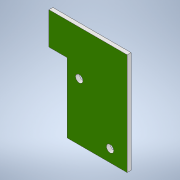
# Autodesk Inventor part: PCB_2_Miras
Saved by Autodesk Inventor 2022 (Build 260153000, 153)
## iProperties
Created: 2023-01-03
Part Number: PCB_2_Miras
Material: Generic
Document SubType Name: Modeling
Designer: Kamil
Density: 1 g/cm^3
Appearance: Default
Author: Kamil
Autodesk Inventor part; units mm, degrees
ref_plane "YZ Plane" through (0, 0, 0) normal (1, 0, 0) x (0, 1, 0)
ref_plane "XZ Plane" through (0, 0, 0) normal (0, 1, 0) x (-1, 0, 0)
ref_plane "XY Plane" through (0, 0, 0) normal (0, 0, 1) x (1, 0, 0)
sketch "Sketch1" plane through (0, 0, 0) normal (0, 0, 1) x (1, 0, 0)
  line L0 (12.5, -5.24) -> (15, -5.24) projected
  line L1 (15, -5.24) -> (15, -10.24) projected
  line L2 (15, -10.24) -> (12.5, -10.24) projected
  arc A0 (12.5, -5.24) -> (12.5, -10.24) centre (12.5, -7.74) ccw projected
  line L3 (-15, -5.24) -> (-12.5, -5.24) projected
  arc A1 (-12.5, -10.24) -> (-12.5, -5.24) centre (-12.5, -7.74) ccw projected
  line L4 (-12.5, -10.24) -> (-15, -10.24) projected
  line L5 (-15, -10.24) -> (-15, -5.24) projected
  circle A2 centre (-7.5, -12.2) radius 1.75 projected
  circle A3 centre (7.5, -12.2) radius 1.75 projected
  line L6 (-37.5, 12.4539) -> (-37.5, -12.4) projected
  line L7 (-34.5, -15.4) -> (34.5, -15.4) projected
  line L8 (37.5, -12.4) -> (37.5, 15.1772) projected
  line L9 (17.8602, 10.1005) -> (17.8602, -0.2) projected
  line L10 (14.8602, -3.2) -> (12.1354, -3.2) projected
  line L11 (10.655, -3.5907) -> (7.417, -5.4279) projected
  line L12 (5.9366, -5.8186) -> (-5.9366, -5.8186) projected
  line L13 (-7.417, -5.4279) -> (-10.655, -3.5907) projected
  line L14 (-12.1354, -3.2) -> (-14.8602, -3.2) projected
  line L15 (-17.8602, -0.2) -> (-17.8602, 10.3433) projected
  line L16 (-13.55, 20.254) -> (-13.55, 16.1005) projected
  line L17 (2.4, 23.254) -> (-10.55, 23.254) projected
  line L18 (2.4, 25.954) -> (2.4, 23.254) projected
  line L19 (4, 25.954) -> (2.4, 25.954) projected
  line L20 (4, 23.254) -> (4, 25.954) projected
  line L21 (5.95, 23.254) -> (4, 23.254) projected
  line L22 (8.95, 16.1005) -> (8.95, 20.254) projected
  line L23 (14.8602, 13.1005) -> (11.95, 13.1005) projected
  line L24 (50, 22.6643) -> (44, 22.6643) projected
  line L25 (44, 22.6643) -> (44, -4.7413) projected
  arc A4 (44, -9.7413) -> (44, -4.7413) centre (44, -7.2413) ccw projected
  line L26 (44, -9.7413) -> (44, -18.8012) projected
  line L27 (44, -18.8012) -> (50, -18.8012) projected
  line L28 (50, -18.8012) -> (50, 22.6643) projected
  line L29 (40.2471, -8.6254) -> (44, -18.8012) projected
  line L30 (44, -9.7413) -> (44, -18.8012) projected
  arc A5 (44, -4.7413) -> (44, -9.7413) centre (44, -7.2413) ccw projected
  line L31 (44, 4.3187) -> (44, -4.7413) projected
  line L32 (44, 4.3187) -> (40.2471, -5.8572) projected
  arc A6 (40.2471, -5.8572) -> (40.2471, -8.6254) centre (44, -7.2413) ccw projected
  line L33 (8.95, 13.1005) -> (37.5, 13.1005)
  line L34 (37.5, 13.1005) -> (37.5, 31.0066)
  line L35 (37.5, 31.0066) -> (8.95, 31.0066)
  line L36 (8.95, 31.0066) -> (8.95, 13.1005)
  line L37 (44, 18.1772) -> (41, 18.1772)
  line L38 (41, 18.1772) -> (41, 7.8033)
  line L39 (41, 7.8033) -> (44, 7.8033)
  line L40 (44, 7.8033) -> (44, 18.1772)
  line L41 (37.5, 31.0066) -> (41, 31.0066)
  line L42 (41, 31.0066) -> (41, 1.9316)
  line L43 (41, 1.9316) -> (37.5, 1.9316)
  line L44 (37.5, 1.9316) -> (37.5, 31.0066)
  line L45 (8.95, 31.0066) -> (41, 31.0066)
  line L46 (41, 31.0066) -> (41, 23.254)
  line L47 (41, 23.254) -> (8.95, 23.254)
  line L48 (8.95, 23.254) -> (8.95, 31.0066)
  line L49 (17.8602, 13.1005) -> (37.5, 13.1005)
  line L50 (37.5, 13.1005) -> (37.5, -15.4)
  line L51 (37.5, -15.4) -> (17.8602, -15.4)
  line L52 (17.8602, -15.4) -> (17.8602, 13.1005)
  line L53 (37.5, -15.4) -> (41, -15.4)
  line L54 (41, -15.4) -> (41, 1.9316)
  line L55 (41, 1.9316) -> (37.5, 1.9316)
  line L56 (37.5, 1.9316) -> (37.5, -15.4)
  arc A7 (-17.7252, -6.9095) -> (-17.704, -4.5096) centre (-17.7146, -5.7096) ccw projected
  line L57 (-17.7252, -6.9095) -> (-18.8252, -6.8998) projected
  arc A8 (-18.8039, -4.4999) -> (-18.8252, -6.8998) centre (-18.8145, -5.6998) ccw projected
  line L58 (-18.8039, -4.4999) -> (-17.704, -4.5096) projected
  circle A9 centre (21.3634, 8.1005) radius 1.5 projected
  arc A10 (-17.5172, 16.5895) -> (-17.496, 18.9894) centre (-17.5066, 17.7895) ccw projected
  line L59 (-17.5172, 16.5895) -> (-18.6172, 16.5993) projected
  arc A11 (-18.5959, 18.9992) -> (-18.6172, 16.5993) centre (-18.6065, 17.7992) ccw projected
  line L60 (-18.5959, 18.9992) -> (-17.496, 18.9894) projected
  circle A12 centre (34, -10.4) radius 1.5 projected
  arc A13 (34.5, -15.4) -> (37.5, -12.4) centre (34.5, -12.4) ccw projected
  arc A14 (37.5, 15.1772) -> (34.5, 18.1772) centre (34.5, 15.1772) ccw projected
  line L61 (34.5, 18.1772) -> (16.4051, 18.1772) projected
  arc A15 (13.4051, 21.1772) -> (16.4051, 18.1772) centre (16.4051, 21.1772) ccw projected
  line L62 (13.4051, 21.1772) -> (13.4051, 28.0066) projected
  arc A16 (13.4051, 28.0066) -> (10.4051, 31.0066) centre (10.4051, 28.0066) ccw projected
  line L63 (10.4051, 31.0066) -> (-18.5665, 31.0066) projected
  arc A17 (-18.5665, 31.0066) -> (-21.5665, 28.0066) centre (-18.5665, 28.0066) ccw projected
  line L64 (-21.5665, 28.0066) -> (-21.5665, 18.4539) projected
  arc A18 (-24.5665, 15.4539) -> (-21.5665, 18.4539) centre (-24.5665, 18.4539) ccw projected
  line L65 (-24.5665, 15.4539) -> (-34.5, 15.4539) projected
  arc A19 (-34.5, 15.4539) -> (-37.5, 12.4539) centre (-34.5, 12.4539) ccw projected
  arc A20 (-37.5, -12.4) -> (-34.5, -15.4) centre (-34.5, -12.4) ccw projected
  arc A21 (-10.655, -3.5907) -> (-12.1354, -3.2) centre (-12.1354, -6.2) ccw projected
  arc A22 (-17.8602, -0.2) -> (-14.8602, -3.2) centre (-14.8602, -0.2) ccw projected
  arc A23 (-15.7051, 13.2219) -> (-17.8602, 10.3433) centre (-14.8602, 10.3433) ccw projected
  arc A24 (-15.7051, 13.2219) -> (-13.55, 16.1005) centre (-16.55, 16.1005) ccw projected
  arc A25 (-10.55, 23.254) -> (-13.55, 20.254) centre (-10.55, 20.254) ccw projected
  arc A26 (8.95, 20.254) -> (5.95, 23.254) centre (5.95, 20.254) ccw projected
  arc A27 (8.95, 16.1005) -> (11.95, 13.1005) centre (11.95, 16.1005) ccw projected
  arc A28 (17.8602, 10.1005) -> (14.8602, 13.1005) centre (14.8602, 10.1005) ccw projected
  arc A29 (14.8602, -3.2) -> (17.8602, -0.2) centre (14.8602, -0.2) ccw projected
  arc A30 (12.1354, -3.2) -> (10.655, -3.5907) centre (12.1354, -6.2) ccw projected
  arc A31 (5.9366, -5.8186) -> (7.417, -5.4279) centre (5.9366, -2.8186) ccw projected
  arc A32 (-7.417, -5.4279) -> (-5.9366, -5.8186) centre (-5.9366, -2.8186) ccw projected
  point P0 (0, 0)
  point P1 (41, -3.8157)
  point P2 (41, -10.6668)
  point P3 (10.4051, 31.0066)
  dimension "d0" = 3
  constraints: 48 end point, 12 parallel, 6 horizontal, 6 perpendicular, 2 point on line
  measures "d0" distance of L39.end L38.end
extrude "Extrusion1" add sketch "Sketch1" along normal blind 3.1 contours L52 L9 L33 L8 A13 L7 | A28 L33 L52 | L8 L34 L47 L42 L38 L43 | L33 L23 A27 L22 L36 L47 L62 A15 L61 A14 L8 | L35 A16 L62 L47 L36 | L33 L36 A27 | L41 L42 L47 L34 | A9 | A12
sketch "Sketch2" plane through (0, 0, 0) normal (0, 0, -1) x (-1, 0, 0)
  line L0 (-17.8602, -15.4) -> (-34.5, -15.4) projected
  line L1 (-17.8602, 10.1005) -> (-17.8602, -15.4) projected
  line L2 (-8.95, 13.1005) -> (-14.8602, 13.1005) projected
  line L3 (-8.95, 31.0066) -> (-8.95, 13.1005) projected
  line L4 (-41, 1.9316) -> (-41, 31.0066) projected
  arc A0 (-16.4051, 18.1772) -> (-13.4051, 21.1772) centre (-16.4051, 21.1772) ccw projected
  line L5 (-34.5, 18.1772) -> (-16.4051, 18.1772) projected
  arc A1 (-34.5, 18.1772) -> (-37.5, 15.1772) centre (-34.5, 15.1772) ccw projected
  line L6 (-37.5, 31.0066) -> (-37.5, 15.1772) projected
  line L7 (-41, 31.0066) -> (-37.5, 31.0066) projected
  line L8 (-37.5, 1.9316) -> (-41, 1.9316) projected
  line L9 (-37.5, -12.4) -> (-37.5, 1.9316) projected
  arc A2 (-37.5, -12.4) -> (-34.5, -15.4) centre (-34.5, -12.4) ccw projected
  arc A3 (-14.8602, 13.1005) -> (-17.8602, 10.1005) centre (-14.8602, 10.1005) ccw projected
  line L10 (-10.4051, 31.0066) -> (-8.95, 31.0066) projected
  arc A4 (-10.4051, 31.0066) -> (-13.4051, 28.0066) centre (-10.4051, 28.0066) ccw projected
  line L11 (-13.4051, 21.1772) -> (-13.4051, 28.0066) projected
  point P0 (0, 0)
extrude "Extrusion2" cut sketch "Sketch2" against normal blind 1.5
sketch "Sketch3" plane through (41, -3.8157, 3.1) normal (1, 0, 0) x (0, 0, -1)
  line L0 (38.317, 76.7923) -> (28.0867, 64.6003) projected
  line L1 (-3.9, -14.9855) -> (-3.9, 26.48) projected
  line L2 (-3.9, -14.9855) -> (7.1, -14.9855) projected
  line L3 (7.1, -14.9855) -> (7.1, 1.1145) projected
  arc A0 (25.2, 19.2145) -> (7.1, 1.1145) centre (25.2, 1.1145) ccw projected
  line L4 (25.2, 19.2145) -> (36.2, 19.2145) projected
  line L5 (1.6, 5.7473) -> (1.6, 34.8223) projected
  line L6 (1.6, 34.8223) -> (0, 34.8223) projected
  line L7 (0, 5.7473) -> (0, 34.8223) projected
  line L8 (0, 0) -> (0, 34.8223) projected
  line L9 (0, 30.197) -> (1.6, 30.197)
  line L10 (28.0867, 30.906) -> (23.6867, 30.906) projected
  line L11 (23.6867, 30.906) -> (23.6867, 44.6714) projected
  line L12 (23.6867, 44.6714) -> (28.0867, 44.6714) projected
  line L13 (28.0867, 44.6714) -> (28.0867, 30.906) projected
  line L14 (28.0867, 64.6003) -> (28.0867, 59.2448) projected
  line L15 (36.2, 19.2145) -> (36.2, 63.075) projected
  line L16 (36.2, 63.075) -> (39.2, 63.075) projected
  line L17 (39.2, 63.075) -> (39.2, 76.4709) projected
  line L18 (23.5929, 59.2448) -> (-3.9, 26.48) projected
  arc A1 (39.2, 76.4709) -> (38.317, 76.7923) centre (38.7, 76.4709) ccw projected
  line L19 (23.5929, 59.2448) -> (28.0867, 59.2448) projected
  line L20 (11.8485, 39.6478) -> (14.4531, 37.4623) projected
  line L21 (14.4531, 37.4623) -> (10.9819, 33.3255) projected
  line L22 (10.9819, 33.3255) -> (8.3773, 35.511) projected
  line L23 (11.8485, 39.6478) -> (8.3773, 35.511) projected
  line L24 (1.6, 5.7473) -> (0, 5.7473) projected
  point P0 (3.1, 3.8157)
  point P1 (36.2, 74.2694)
  constraints: 2 end point, 2 point on line, 1 perpendicular
extrude "Extrusion3" cut sketch "Sketch3" against normal through all contours L18 L7 L6 L5 | L5 L9 L7 L18
sketch "Sketch4" plane through (0, 0, 3.1) normal (0, 0, 1) x (1, 0, 0)
  line L0 (31.7, -15.7) -> (31.7, 9.3) projected
  line L1 (13.4051, 26.3813) -> (8.95, 26.3813) projected
  line L2 (8.95, 26.3813) -> (8.95, 13.1005) projected
  line L3 (8.95, 13.1005) -> (14.8602, 13.1005) projected
  line L4 (17.8602, 10.1005) -> (17.8602, -15.4) projected
  line L5 (17.8602, -15.4) -> (34.5, -15.4) projected
  line L6 (41, 1.9316) -> (41, 26.3813) projected
  line L7 (41, -15.4) -> (41, -10.6668) projected
  line L8 (41, -3.8157) -> (41, -10.6668)
  arc A0 (17.8602, 10.1005) -> (14.8602, 13.1005) centre (14.8602, 10.1005) ccw projected
  arc A1 (34.5, -15.4) -> (37.5, -12.4) centre (34.5, -12.4) ccw projected
  line L9 (37.5, -12.4) -> (37.5, 1.9316) projected
  line L10 (37.5, 1.9316) -> (41, 1.9316) projected
  line L11 (41, 26.3813) -> (37.5, 26.3813) projected
  line L12 (37.5, 26.3813) -> (37.5, 15.1772) projected
  arc A2 (37.5, 15.1772) -> (34.5, 18.1772) centre (34.5, 15.1772) ccw projected
  line L13 (34.5, 18.1772) -> (16.4051, 18.1772) projected
  arc A3 (13.4051, 21.1772) -> (16.4051, 18.1772) centre (16.4051, 21.1772) ccw projected
  line L14 (13.4051, 21.1772) -> (13.4051, 26.3813) projected
  point P0 (0, 0)
  constraints: 2 end point
extrude "Extrusion4" [suppressed]
sketch "Sketch5" plane through (0, 0, 3.1) normal (0, 0, 1) x (1, 0, 0)
  line L0 (13.4051, 26.3813) -> (8.95, 26.3813) projected
  line L1 (8.95, 26.3813) -> (8.95, 13.1005) projected
  line L2 (8.95, 13.1005) -> (14.8602, 13.1005) projected
  line L3 (17.8602, 10.1005) -> (17.8602, -15.4) projected
  line L4 (17.8602, -15.4) -> (34.5, -15.4) projected
  line L5 (15, 8.3373) -> (15, -1.2152) projected
  line L6 (8.95, 13.1005) -> (17.8602, 13.1005) projected
  line L7 (17.8602, 13.1005) -> (16.3634, 13.1005)
  line L8 (16.3634, 13.1005) -> (16.3634, -15.4)
  line L9 (16.3634, -15.4) -> (17.8602, -15.4)
  line L10 (17.8602, -15.4) -> (17.8602, 13.1005)
  arc A0 (17.8602, 10.1005) -> (14.8602, 13.1005) centre (14.8602, 10.1005) ccw projected
  arc A1 (34.5, -15.4) -> (37.5, -12.4) centre (34.5, -12.4) ccw projected
  line L11 (37.5, -12.4) -> (37.5, 1.9316) projected
  line L12 (37.5, 1.9316) -> (41, 1.9316) projected
  line L13 (41, 1.9316) -> (41, 26.3813) projected
  line L14 (41, 26.3813) -> (37.5, 26.3813) projected
  line L15 (37.5, 26.3813) -> (37.5, 15.1772) projected
  arc A2 (37.5, 15.1772) -> (34.5, 18.1772) centre (34.5, 15.1772) ccw projected
  line L16 (34.5, 18.1772) -> (16.4051, 18.1772) projected
  arc A3 (13.4051, 21.1772) -> (16.4051, 18.1772) centre (16.4051, 21.1772) ccw projected
  line L17 (13.4051, 21.1772) -> (13.4051, 26.3813) projected
  point P0 (0, 0)
  point P1 (16.3634, 12.6967)
  constraints: 8 end point, 2 parallel, 1 horizontal, 1 perpendicular
extrude "Extrusion5" add sketch "Sketch5" against normal blind 1.6 contours A0 L3 L9 L8
sketch "Sketch6" plane through (0, 0, 3.1) normal (0, 0, 1) x (1, 0, 0)
  line L0 (13.4051, 26.3813) -> (8.95, 26.3813) projected
  line L1 (8.95, 26.3813) -> (8.95, 13.1005) projected
  line L2 (8.95, 13.1005) -> (14.8602, 13.1005) projected
  line L3 (16.3634, 12.6967) -> (16.3634, -15.4) projected
  line L4 (16.3634, -15.4) -> (34.5, -15.4) projected
  line L5 (16.3634, -15.4) -> (41, -15.4) projected
  line L6 (28.6817, -15.4) -> (28.6817, 26.3813)
  line L7 (41, 26.3813) -> (8.95, 26.3813) projected
  line L8 (28.6817, -15.4) -> (28.6817, -9.9)
  line L9 (28.6817, 26.3813) -> (28.6817, 20.8813)
  line L10 (16.3634, 13.1005) -> (41, 13.1005)
  line L11 (41, -15.4) -> (41, 26.3813) projected
  line L12 (16.3634, 13.1005) -> (21.3634, 13.1005)
  line L13 (21.3634, 13.1005) -> (21.3634, 8.1005)
  line L14 (21.3634, 8.1005) -> (16.3634, 8.1005)
  line L15 (16.3634, 8.1005) -> (16.3634, 13.1005)
  line L16 (41, -15.4) -> (36, -15.4)
  line L17 (36, -15.4) -> (36, -10.4)
  line L18 (36, -10.4) -> (41, -10.4)
  line L19 (41, -10.4) -> (41, -15.4)
  circle A0 centre (21.3634, 8.1005) radius 1.5
  circle A1 centre (36, -10.4) radius 1.5
  arc A2 (16.3634, 12.6967) -> (14.8602, 13.1005) centre (14.8602, 10.1005) ccw projected
  arc A3 (34.5, -15.4) -> (37.5, -12.4) centre (34.5, -12.4) ccw projected
  line L20 (37.5, -12.4) -> (37.5, 1.9316) projected
  line L21 (37.5, 1.9316) -> (41, 1.9316) projected
  line L22 (41, 1.9316) -> (41, 26.3813) projected
  line L23 (41, 26.3813) -> (37.5, 26.3813) projected
  line L24 (37.5, 26.3813) -> (37.5, 15.1772) projected
  arc A4 (37.5, 15.1772) -> (34.5, 18.1772) centre (34.5, 15.1772) ccw projected
  line L25 (34.5, 18.1772) -> (16.4051, 18.1772) projected
  arc A5 (13.4051, 21.1772) -> (16.4051, 18.1772) centre (16.4051, 21.1772) ccw projected
  line L26 (13.4051, 21.1772) -> (13.4051, 26.3813) projected
  point P0 (0, 0)
  dimension "d11" = 5.5
  dimension "d12" = 5.5
  dimension "d13" = 5
  dimension "d14" = 5
  dimension "d15" = 5
  dimension "d16" = 5
  dimension "d17" = 3
  dimension "d18" = 3
  constraints: 24 end point, 4 parallel, 4 point on line, 3 perpendicular, 2 centre point, 2 coincident, 2 horizontal, 1 midpoint
  measures "d11" distance of L6.start L8.end
  measures "d12" distance of L6.end L9.end
  measures "d13" distance of L13.end L14.end
  measures "d14" distance of L12.end L13.end
  measures "d15" distance of L17.end L18.end
  measures "d16" distance of L16.end L17.end
  measures "d17" diameter of A0
  measures "d18" diameter of A1
extrude "Extrusion6" cut sketch "Sketch6" against normal blind 1.6 contours A0 L13 L14 | L14 L13 A0 | A1 L17 L18 | L18 L17 A1
sketch "Sketch8" plane through (0, 0, 3.1) normal (0, 0, 1) x (1, 0, 0)
  circle A0 centre (36, -10.4) radius 1.5 projected
  circle A1 centre (21.3634, 8.1005) radius 1.5 projected
  line L0 (13.4051, 26.3813) -> (8.95, 26.3813) projected
  line L1 (8.95, 26.3813) -> (8.95, 13.1005) projected
  line L2 (8.95, 13.1005) -> (14.8602, 13.1005) projected
  line L3 (16.3634, 12.6967) -> (16.3634, -15.4) projected
  line L4 (16.3634, -15.4) -> (34.5, -15.4) projected
  line L5 (36, -10.4) -> (34, -10.4)
  circle A2 centre (34, -10.4) radius 1.5
  arc A3 (16.3634, 12.6967) -> (14.8602, 13.1005) centre (14.8602, 10.1005) ccw projected
  arc A4 (34.5, -15.4) -> (37.5, -12.4) centre (34.5, -12.4) ccw projected
  line L6 (37.5, -12.4) -> (37.5, -10.4) projected
  line L7 (37.5, -10.4) -> (37.5, 1.9316) projected
  line L8 (37.5, 1.9316) -> (41, 1.9316) projected
  line L9 (41, 1.9316) -> (41, 26.3813) projected
  line L10 (41, 26.3813) -> (37.5, 26.3813) projected
  line L11 (37.5, 26.3813) -> (37.5, 15.1772) projected
  arc A5 (37.5, 15.1772) -> (34.5, 18.1772) centre (34.5, 15.1772) ccw projected
  line L12 (34.5, 18.1772) -> (16.4051, 18.1772) projected
  arc A6 (13.4051, 21.1772) -> (16.4051, 18.1772) centre (16.4051, 21.1772) ccw projected
  line L13 (13.4051, 21.1772) -> (13.4051, 26.3813) projected
  point P0 (0, 0)
  dimension "d21" = 2
  constraints: 2 end point, 1 centre point, 1 coincident, 1 horizontal, 1 horizontal alignment
  measures "d21" distance of L5.start L5.end
extrude "Extrusion7" add sketch "Sketch8" against normal blind 1.6 contours A0 A2 | A2 L5 A0 | A0 L5 A2 picked at (36.8202, -10.286)
extrude "Extrusion8" cut sketch "Sketch8" against normal blind 1.6 contours A2 L5 A0 | A0 A2 | A0 L5 A2 picked at (33.174, -10.4)
sketch "Sketch9" plane through (0, 0, 3.1) normal (0, 0, 1) x (1, 0, 0)
  circle A0 centre (34, -10.4) radius 1.5 projected
  line L0 (13.4051, 26.3813) -> (8.95, 26.3813) projected
  line L1 (8.95, 26.3813) -> (8.95, 13.1005) projected
  line L2 (8.95, 13.1005) -> (14.8602, 13.1005) projected
  arc A1 (16.3634, 12.6967) -> (14.8602, 13.1005) centre (14.8602, 10.1005) ccw projected
  line L3 (16.3634, 12.6967) -> (16.3634, -15.4) projected
  line L4 (16.3634, -15.4) -> (34.5, -15.4) projected
  arc A2 (34.5, -15.4) -> (37.5, -12.4) centre (34.5, -12.4) ccw projected
  line L5 (37.5, -12.4) -> (37.5, 1.9316) projected
  line L6 (37.5, 1.9316) -> (41, 1.9316) projected
  line L7 (41, 1.9316) -> (41, 26.3813) projected
  line L8 (41, 26.3813) -> (37.5, 26.3813) projected
  line L9 (37.5, 26.3813) -> (37.5, 15.1772) projected
  arc A3 (37.5, 15.1772) -> (34.5, 18.1772) centre (34.5, 15.1772) ccw projected
  line L10 (34.5, 18.1772) -> (16.4051, 18.1772) projected
  arc A4 (13.4051, 21.1772) -> (16.4051, 18.1772) centre (16.4051, 21.1772) ccw projected
  line L11 (13.4051, 21.1772) -> (13.4051, 26.3813) projected
  circle A5 centre (21.3634, 8.1005) radius 1.5 projected
  line L12 (8.95, 13.1005) -> (41, 13.1005)
  line L13 (41, 13.1005) -> (41, 26.3813)
  line L14 (41, 26.3813) -> (8.95, 26.3813)
  line L15 (8.95, 26.3813) -> (8.95, 13.1005)
  point P0 (0, 0)
  constraints: 8 end point, 2 parallel, 1 horizontal, 1 perpendicular
extrude "Extrusion9" add sketch "Sketch9" against normal blind 1.6 contours L14 L9 A3 L10 A4 L11
sketch "Sketch10" plane through (0, 0, 3.1) normal (0, 0, 1) x (1, 0, 0)
  circle A0 centre (34, -10.4) radius 1.5 projected
  line L0 (41, 26.3813) -> (8.95, 26.3813) projected
  line L1 (8.95, 26.3813) -> (8.95, 13.1005) projected
  line L2 (8.95, 13.1005) -> (14.8602, 13.1005) projected
  arc A1 (16.3634, 12.6967) -> (14.8602, 13.1005) centre (14.8602, 10.1005) ccw projected
  line L3 (16.3634, 12.6967) -> (16.3634, -15.4) projected
  line L4 (16.3634, -15.4) -> (34.5, -15.4) projected
  arc A2 (34.5, -15.4) -> (37.5, -12.4) centre (34.5, -12.4) ccw projected
  line L5 (37.5, -12.4) -> (37.5, 1.9316) projected
  line L6 (37.5, 1.9316) -> (41, 1.9316) projected
  line L7 (41, 1.9316) -> (41, 26.3813) projected
  circle A3 centre (21.3634, 8.1005) radius 1.5 projected
  line L8 (41, 1.9316) -> (37.5, 1.9316)
  line L9 (37.5, 1.9316) -> (37.5, -15.4)
  line L10 (37.5, -15.4) -> (41, -15.4)
  line L11 (41, -15.4) -> (41, 1.9316)
  arc A4 (34.5, -15.4) -> (37.5, -12.4) centre (34.5, -12.4) ccw projected
  line L12 (37.5, -15.4) -> (34.5, -15.4)
  line L13 (34.5, -15.4) -> (34.5, -12.4)
  line L14 (34.5, -12.4) -> (37.5, -12.4)
  line L15 (37.5, -12.4) -> (37.5, -15.4)
  point P0 (0, 0)
  constraints: 16 end point, 4 parallel, 2 horizontal, 2 perpendicular
extrude "Extrusion10" add sketch "Sketch10" against normal blind 1.6 contours L11 L10 L9 L5 L6 | L9 L12 A2 | A2 L13 L14
body "Solid1"
